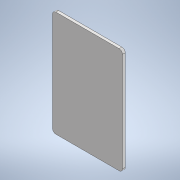
# Autodesk Inventor part: LimitSwitch Con Lid
Saved by Autodesk Inventor 2020 (Build 240168000, 168)
## iProperties
Created: 2019-04-18
Part Number: LimitSwitch Con Lid
Material: Generic
Document SubType Name: Modeling
Designer: Parker
Density: 1 g/cm^3
Appearance: Default
Author: Parker
Autodesk Inventor part; units mm, degrees
ref_plane "YZ Plane" through (0, 0, 0) normal (1, 0, 0) x (0, 1, 0)
ref_plane "XZ Plane" through (0, 0, 0) normal (0, 1, 0) x (-1, 0, 0)
ref_plane "XY Plane" through (0, 0, 0) normal (0, 0, 1) x (1, 0, 0)
sketch "Sketch1" plane through (0, 0, 0) normal (0, 0, 1) x (1, 0, 0)
  line L0 (11.5, 20) -> (-11.5, 20) projected
  arc A0 (-11.5, 20) -> (-13.5, 18) centre (-11.5, 18) ccw projected
  line L1 (-13.5, 18) -> (-13.5, -18) projected
  arc A1 (-13.5, -18) -> (-11.5, -20) centre (-11.5, -18) ccw projected
  line L2 (-11.5, -20) -> (11.5, -20) projected
  arc A2 (11.5, -20) -> (13.5, -18) centre (11.5, -18) ccw projected
  line L3 (13.5, -18) -> (13.5, 18) projected
  arc A3 (13.5, 18) -> (11.5, 20) centre (11.5, 18) ccw projected
  arc A4 (-12.7, -18) -> (-11.5, -19.2) centre (-11.5, -18) ccw projected
  line L4 (-12.7, -18) -> (-12.7, 18) projected
  arc A5 (-11.5, 19.2) -> (-12.7, 18) centre (-11.5, 18) ccw projected
  line L5 (-11.5, 19.2) -> (11.5, 19.2) projected
  arc A6 (12.7, 18) -> (11.5, 19.2) centre (11.5, 18) ccw projected
  line L6 (12.7, 18) -> (12.7, -18) projected
  arc A7 (11.5, -19.2) -> (12.7, -18) centre (11.5, -18) ccw projected
  line L7 (11.5, -19.2) -> (-11.5, -19.2) projected
  point P0 (0, 0)
extrude "Extrusion1" add sketch "Sketch1" against normal blind 1 contours L4 A5 L5 A6 L6 A7 L7 A4
sketch "Sketch2" plane through (0, 0, -1) normal (0, 0, -1) x (-1, 0, 0)
  line L0 (-7.8847, 4.0217) -> (7.8847, 4.0217)
  line L1 (7.8847, 4.0217) -> (7.8847, 0)
  line L2 (7.8847, 0) -> (-7.8847, 0)
  line L3 (-7.8847, 0) -> (-7.8847, 4.0217)
  line L4 (-7.8847, 4.0217) -> (7.8847, 0) construction
  line L5 (7.8847, 4.0217) -> (-7.8847, 0) construction
  point P0 (0, 0)
  point P1 (0, 2.0108)
  constraints: 12 end point, 2 midpoint, 2 parallel, 1 horizontal, 1 perpendicular
extrude "Extrusion2" add sketch "Sketch2" along normal blind 0.8
sketch "Sketch3" plane through (0, 0, 0) normal (0, 0, 1) x (1, 0, 0)
  circle A0 centre (0, 6.524) radius 9.0102
  line L0 (1.757, 4.8742) -> (7.0929, 9.7934)
  line L1 (3.0889, 4.4699) -> (7.5372, 8.5709)
  line L2 (-4.4419, 5.5016) -> (-1.81, -1.0736)
  line L3 (-2.9706, 5.055) -> (-0.4373, -1.274)
  line L4 (-7.8102, 6.524) -> (-4.4419, 5.5016)
  line L5 (-2.9706, 5.055) -> (6.4925, 2.1827)
  arc A1 (-7.8102, 6.524) -> (-1.81, -1.0736) centre (0, 6.524) ccw
  line L6 (-7.7136, 7.7487) -> (1.757, 4.8742)
  line L7 (3.0889, 4.4699) -> (7.0929, 3.2545)
  arc A2 (7.0929, 9.7934) -> (-7.7136, 7.7487) centre (0, 6.524) ccw
  arc A3 (-0.4373, -1.274) -> (6.4925, 2.1827) centre (0, 6.524) ccw
  arc A4 (7.0929, 3.2545) -> (7.5372, 8.5709) centre (0, 6.524) ccw
  dimension "d16" = 1.2
  dimension "d17" = 1.2
  constraints: 16 end point, 8 point on circle, 6 parallel, 5 centre point
  measures "d16" distance between parallel lines of L0 L1
  measures "d17" distance between parallel lines of L2 L3
extrude "Extrusion3" cut sketch "Sketch3" against normal blind 0.2
sketch "Sketch4" plane through (0, 0, 0) normal (0, 0, 1) x (1, 0, 0)
  line L0 (-8.3854, -4.5453) -> (2.4185, -4.5453) construction
  line L1 (2.4185, -4.5453) -> (2.4185, -8.8273) construction
  line L2 (2.4185, -8.8273) -> (-8.3854, -8.8273) construction
  line L3 (-8.3854, -8.8273) -> (-8.3854, -4.5453) construction
  line L4 (-7.9406, -12.5453) -> (-7.9406, -4.5453)
  line L5 (-7.9406, -4.5453) -> (-4.8392, -4.5453)
  spline S0 degree 2 poles (-4.8392, -4.5453) (-3.7754, -4.5453) (-2.6754, -5.4649) (-2.5071, -6.4927) knots 0 0 0 1 2 2 2
  spline S1 degree 2 poles (-2.5071, -6.4927) (-2.4651, -6.8233) (-2.453, -7.0096) (-2.453, -7.1358) knots 0 0 0 1 2 2 2
  spline S2 degree 2 poles (-2.453, -7.1358) (-2.453, -8.2478) (-3.8174, -9.4799) (-5.0496, -9.4799) knots 0 0 0 1 2 2 2
  line L6 (-5.0496, -9.4799) -> (-5.8189, -9.4799)
  line L7 (-5.8189, -9.4799) -> (-5.8189, -12.5453)
  line L8 (-5.8189, -12.5453) -> (-7.9406, -12.5453)
  spline S3 degree 2 poles (-5.3561, -7.9713) (-5.1458, -7.9713) (-4.713, -7.6347) (-4.6469, -7.3041) knots 0 0 0 1 2 2 2
  spline S4 degree 2 poles (-4.6469, -7.3041) (-4.6108, -7.1358) (-4.6108, -6.9916) knots 0 0 0 1 1 1
  spline S5 degree 2 poles (-4.6108, -6.9916) (-4.6108, -6.5648) (-5.0195, -6.066) (-5.3321, -6.066) knots 0 0 0 1 2 2 2
  line L9 (-5.3321, -6.066) -> (-5.8189, -6.066)
  line L10 (-5.8189, -6.066) -> (-5.8189, -7.9713)
  line L11 (-5.8189, -7.9713) -> (-5.3561, -7.9713)
  line L12 (-2.0203, -12.5453) -> (-2.0203, -4.5453)
  line L13 (-2.0203, -4.5453) -> (2.686, -4.5453)
  line L14 (2.686, -4.5453) -> (2.686, -6.2222)
  line L15 (2.686, -6.2222) -> (0.1014, -6.2222)
  line L16 (0.1014, -6.2222) -> (0.1014, -7.6708)
  line L17 (0.1014, -7.6708) -> (2.5357, -7.6708)
  line L18 (2.5357, -7.6708) -> (2.5357, -9.2696)
  line L19 (2.5357, -9.2696) -> (0.1014, -9.2696)
  line L20 (0.1014, -9.2696) -> (0.1014, -10.8684)
  line L21 (0.1014, -10.8684) -> (2.7761, -10.8684)
  line L22 (2.7761, -10.8684) -> (2.7761, -12.5453)
  line L23 (2.7761, -12.5453) -> (-2.0203, -12.5453)
  line L24 (3.4252, -12.5453) -> (3.4252, -4.5453)
  line L25 (3.4252, -4.5453) -> (6.5267, -4.5453)
  spline S6 degree 2 poles (6.5267, -4.5453) (7.5905, -4.5453) (8.6905, -5.4649) (8.8588, -6.4927) knots 0 0 0 1 2 2 2
  spline S7 degree 2 poles (8.8588, -6.4927) (8.9008, -6.8233) (8.9129, -7.0096) (8.9129, -7.1358) knots 0 0 0 1 2 2 2
  spline S8 degree 2 poles (8.9129, -7.1358) (8.9129, -8.2478) (7.5485, -9.4799) (6.3163, -9.4799) knots 0 0 0 1 2 2 2
  line L26 (6.3163, -9.4799) -> (5.547, -9.4799)
  line L27 (5.547, -9.4799) -> (5.547, -12.5453)
  line L28 (5.547, -12.5453) -> (3.4252, -12.5453)
  spline S9 degree 2 poles (6.0098, -7.9713) (6.2201, -7.9713) (6.6529, -7.6347) (6.719, -7.3041) knots 0 0 0 1 2 2 2
  spline S10 degree 2 poles (6.719, -7.3041) (6.7551, -7.1358) (6.7551, -6.9916) knots 0 0 0 1 1 1
  spline S11 degree 2 poles (6.7551, -6.9916) (6.7551, -6.5648) (6.3464, -6.066) (6.0338, -6.066) knots 0 0 0 1 2 2 2
  line L29 (6.0338, -6.066) -> (5.547, -6.066)
  line L30 (5.547, -6.066) -> (5.547, -7.9713)
  line L31 (5.547, -7.9713) -> (6.0098, -7.9713)
  point P0 (0, 0)
  constraints: 2 other
extrude "Extrusion4" cut sketch "Sketch4" against normal blind 0.2
body "Solid1"
